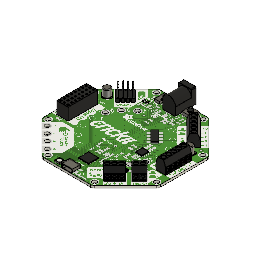
3093 Crickit CPX (Autodesk Fusion 360 design; units mm, degrees)
Autodesk Fusion 360 part; units mm, degrees
note: some values were not read from the file. Chosen so that the rebuilt part matches the saved one: which bodies a step acts on; which pieces of a blend or face edit are solid. Set by a fixed rule: which sketch regions a step uses.
(part 1 of 2)
sketch "cpx crickit" plane through (0, 0, 0) normal (0, 0, 1) x (1, 0, 0)
  arc A0 (-0.865, 37.0412) -> (-1.115, 36.7912) centre (-0.865, 36.7912) ccw
  arc A1 (2.385, 36.7912) -> (2.135, 37.0412) centre (2.135, 36.7912) ccw
  line L0 (16.3469, -40.64) -> (-16.3469, -40.64)
  line L1 (-4.3642, 34.692) -> (-3.915, 34.692)
  line L2 (-3.915, 31.692) -> (-4.3642, 31.692)
  arc A2 (-4.3642, 34.692) -> (-4.6142, 34.442) centre (-4.3642, 34.442) ccw
  arc A3 (-0.865, 30.7912) -> (-1.115, 30.592) centre (-0.8904, 30.5666) ccw
  arc A4 (40.64, 16.3469) -> (39.8961, 18.143) centre (38.1, 16.3469) ccw
  line L3 (-0.865, 37.0412) -> (2.135, 37.0412)
  line L4 (18.143, 39.8961) -> (39.8961, 18.143)
  arc A5 (2.135, 29.8928) -> (2.385, 30.092) centre (2.1604, 30.1174) ccw
  circle A6 centre (-9.779, 33.679) radius 0.5
  arc A7 (2.385, 30.592) -> (2.135, 30.7912) centre (2.1604, 30.5666) ccw
  arc A8 (-3.7158, 34.4674) -> (-3.915, 34.692) centre (-3.9277, 34.4801) ccw
  line L5 (-18.143, -39.8961) -> (-39.8961, -18.143)
  line L6 (2.135, 29.8928) -> (-0.865, 29.8928)
  arc A9 (18.143, 39.8961) -> (16.3469, 40.64) centre (16.3469, 38.1) ccw
  arc A10 (-3.915, 31.692) -> (-3.7158, 31.9674) centre (-3.9531, 31.9293) ccw
  line L7 (-1.115, 30.092) -> (-1.115, 30.592)
  line L8 (-0.865, 30.7912) -> (2.135, 30.7912)
  arc A11 (-4.6142, 31.942) -> (-4.3642, 31.692) centre (-4.3642, 31.942) ccw
  arc A12 (-1.115, 30.092) -> (-0.865, 29.8928) centre (-0.8904, 30.1174) ccw
  line L9 (4.05, -37.922) -> (4.05, -38.522)
  line L10 (-3.7158, 34.4674) -> (-3.7158, 31.9674)
  line L11 (-3.7, -37.572) -> (-3.5, -37.572)
  line L12 (2.385, 36.7912) -> (2.385, 36.3928)
  line L13 (40.64, 16.3469) -> (40.64, -16.3469)
  arc A13 (-4.05, -38.472) -> (-3.7, -38.872) centre (-3.675, -38.497) ccw
  arc A14 (3.6, -38.872) -> (4.05, -38.522) centre (3.65, -38.472) ccw
  circle A15 centre (-9.779, 36.679) radius 0.5
  arc A16 (-3.5, -38.872) -> (-3.15, -38.472) centre (-3.525, -38.497) ccw
  line L14 (-4.6142, 31.942) -> (-4.6142, 34.442)
  circle A17 centre (-1.95, -36.322) radius 0.35
  line L15 (-3.5, -38.872) -> (-3.7, -38.872)
  line L16 (-1.115, 36.3928) -> (-1.115, 36.7912)
  circle A18 centre (1.95, -36.322) radius 0.35
  line L17 (-39.8961, 18.143) -> (-18.143, 39.8961)
  arc A19 (2.135, 36.1428) -> (2.385, 36.3928) centre (2.135, 36.3928) ccw
  line L18 (-40.64, -16.3469) -> (-40.64, 16.3469)
  line L19 (3.15, -38.522) -> (3.15, -37.922)
  arc A20 (-39.8961, 18.143) -> (-40.64, 16.3469) centre (-38.1, 16.3469) ccw
  arc A21 (3.15, -38.522) -> (3.6, -38.872) centre (3.55, -38.472) ccw
  line L20 (2.135, 36.1428) -> (-0.865, 36.1428)
  line L21 (2.385, 30.592) -> (2.385, 30.092)
  arc A22 (-3.7, -37.572) -> (-4.05, -37.922) centre (-3.7, -37.922) ccw
  line L22 (-4.05, -38.472) -> (-4.05, -37.922)
  line L23 (39.8961, -18.143) -> (18.143, -39.8961)
  arc A23 (-1.115, 36.3928) -> (-0.865, 36.1428) centre (-0.865, 36.3928) ccw
  arc A24 (4.05, -37.922) -> (3.6, -37.572) centre (3.65, -37.972) ccw
  arc A25 (16.3469, -40.64) -> (18.143, -39.8961) centre (16.3469, -38.1) ccw
  line L24 (-16.3469, 40.64) -> (16.3469, 40.64)
  arc A26 (39.8961, -18.143) -> (40.64, -16.3469) centre (38.1, -16.3469) ccw
  arc A27 (-3.15, -37.922) -> (-3.5, -37.572) centre (-3.5, -37.922) ccw
  line L25 (-3.15, -37.922) -> (-3.15, -38.472)
  arc A28 (-16.3469, 40.64) -> (-18.143, 39.8961) centre (-16.3469, 38.1) ccw
  arc A29 (-18.143, -39.8961) -> (-16.3469, -40.64) centre (-16.3469, -38.1) ccw
  arc A30 (3.6, -37.572) -> (3.15, -37.922) centre (3.55, -37.972) ccw
  arc A31 (-40.64, -16.3469) -> (-39.8961, -18.143) centre (-38.1, -16.3469) ccw
  arc A32 (2.3241, -8.89) -> (1.4859, -8.89) centre (1.905, -8.89) ccw
  line L26 (1.985, 36.592) -> (-0.715, 36.592)
  arc A33 (16.129, 36.715) -> (16.129, 38.723) centre (16.129, 37.719) ccw
  arc A34 (-16.129, 38.723) -> (-16.129, 36.715) centre (-16.129, 37.719) ccw
  arc A35 (-16.129, 36.715) -> (-16.129, 38.723) centre (-16.129, 37.719) ccw
  arc A36 (3.3, -35.095) -> (3.3, -35.749) centre (3.3, -35.422) ccw
  arc A37 (37.719, 15.125) -> (37.719, 17.133) centre (37.719, 16.129) ccw
  arc A38 (-16.129, -38.723) -> (-16.129, -36.715) centre (-16.129, -37.719) ccw
  line L27 (-2.3935, -39.4285) -> (-2.3935, -37.0155)
  line L28 (2.3935, -39.4285) -> (4.8065, -39.4285)
  line L29 (-4.8065, -37.0155) -> (-4.8065, -39.4285)
  arc A39 (16.129, -38.723) -> (16.129, -36.715) centre (16.129, -37.719) ccw
  arc A40 (-16.129, -38.723) -> (-16.129, -36.715) centre (-16.129, -37.719) ccw
  arc A41 (37.719, 15.125) -> (37.719, 17.133) centre (37.719, 16.129) ccw
  line L30 (4.8065, -37.0155) -> (2.3935, -37.0155)
  arc A42 (-37.719, -17.133) -> (-37.719, -15.125) centre (-37.719, -16.129) ccw
  arc A43 (-37.719, -17.133) -> (-37.719, -15.125) centre (-37.719, -16.129) ccw
  arc A44 (1.985, 35.917) -> (1.985, 37.267) centre (1.985, 36.592) ccw
  arc A45 (16.129, 36.715) -> (16.129, 38.723) centre (16.129, 37.719) ccw
  line L31 (-3.3, -35.422) -> (-4.608, -35.422)
  arc A46 (37.719, -17.133) -> (37.719, -15.125) centre (37.719, -16.129) ccw
  line L32 (-2.3935, -37.0155) -> (-4.8065, -37.0155)
  arc A47 (37.719, -15.125) -> (37.719, -17.133) centre (37.719, -16.129) ccw
  line L33 (3.3, -35.422) -> (4.608, -35.422)
  arc A48 (-4.608, -35.095) -> (-4.608, -35.749) centre (-4.608, -35.422) ccw
  line L34 (2.3935, -39.4285) -> (4.8065, -39.4285)
  line L35 (-3.3, -35.422) -> (-4.608, -35.422)
  arc A49 (-16.129, 36.715) -> (-16.129, 38.723) centre (-16.129, 37.719) ccw
  arc A50 (16.129, 38.723) -> (16.129, 36.715) centre (16.129, 37.719) ccw
  arc A51 (-3.3, -35.749) -> (-3.3, -35.095) centre (-3.3, -35.422) ccw
  arc A52 (-3.3, -35.749) -> (-3.3, -35.095) centre (-3.3, -35.422) ccw
  arc A53 (-16.129, -36.715) -> (-16.129, -38.723) centre (-16.129, -37.719) ccw
  arc A54 (-0.715, 31.017) -> (-0.715, 29.667) centre (-0.715, 30.342) ccw
  line L36 (2.3935, -37.0155) -> (2.3935, -39.4285)
  line L37 (2.3935, -37.0155) -> (2.3935, -39.4285)
  arc A55 (37.719, 17.133) -> (37.719, 15.125) centre (37.719, 16.129) ccw
  line L38 (1.985, 36.592) -> (-0.715, 36.592)
  arc A56 (1.985, 29.667) -> (1.985, 31.017) centre (1.985, 30.342) ccw
  arc A57 (16.129, 38.723) -> (16.129, 36.715) centre (16.129, 37.719) ccw
  line L39 (4.8065, -37.0155) -> (2.3935, -37.0155)
  line L40 (-2.3935, -39.4285) -> (-2.3935, -37.0155)
  arc A58 (-3.49, 34.542) -> (-4.84, 34.542) centre (-4.165, 34.542) ccw
  line L41 (-4.8065, -39.4285) -> (-2.3935, -39.4285)
  arc A59 (-37.719, -15.125) -> (-37.719, -17.133) centre (-37.719, -16.129) ccw
  arc A60 (-37.719, 17.133) -> (-37.719, 15.125) centre (-37.719, 16.129) ccw
  arc A61 (-0.715, 31.017) -> (-0.715, 29.667) centre (-0.715, 30.342) ccw
  line L42 (-4.165, 34.542) -> (-4.165, 31.842)
  arc A62 (-4.84, 31.842) -> (-3.49, 31.842) centre (-4.165, 31.842) ccw
  arc A63 (-37.719, 15.125) -> (-37.719, 17.133) centre (-37.719, 16.129) ccw
  line L43 (4.8065, -39.4285) -> (4.8065, -37.0155)
  line L44 (-4.165, 34.542) -> (-4.165, 31.842)
  line L45 (-4.8065, -39.4285) -> (-2.3935, -39.4285)
  arc A64 (1.985, 35.917) -> (1.985, 37.267) centre (1.985, 36.592) ccw
  arc A65 (-37.719, 17.133) -> (-37.719, 15.125) centre (-37.719, 16.129) ccw
  arc A66 (37.719, 17.133) -> (37.719, 15.125) centre (37.719, 16.129) ccw
  arc A67 (16.129, -36.715) -> (16.129, -38.723) centre (16.129, -37.719) ccw
  arc A68 (1.4859, -8.89) -> (2.3241, -8.89) centre (1.905, -8.89) ccw
  arc A69 (-4.608, -35.095) -> (-4.608, -35.749) centre (-4.608, -35.422) ccw
  arc A70 (4.608, -35.749) -> (4.608, -35.095) centre (4.608, -35.422) ccw
  arc A71 (16.129, -36.715) -> (16.129, -38.723) centre (16.129, -37.719) ccw
  arc A72 (-16.129, 38.723) -> (-16.129, 36.715) centre (-16.129, 37.719) ccw
  line L46 (-2.3935, -37.0155) -> (-4.8065, -37.0155)
  arc A73 (37.719, -15.125) -> (37.719, -17.133) centre (37.719, -16.129) ccw
  arc A74 (3.3, -35.095) -> (3.3, -35.749) centre (3.3, -35.422) ccw
  arc A75 (-0.715, 37.267) -> (-0.715, 35.917) centre (-0.715, 36.592) ccw
  line L47 (1.985, 30.342) -> (-0.715, 30.342)
  arc A76 (-37.719, 15.125) -> (-37.719, 17.133) centre (-37.719, 16.129) ccw
  arc A77 (16.129, -38.723) -> (16.129, -36.715) centre (16.129, -37.719) ccw
  arc A78 (-3.49, 34.542) -> (-4.84, 34.542) centre (-4.165, 34.542) ccw
  line L48 (-4.8065, -37.0155) -> (-4.8065, -39.4285)
  arc A79 (37.719, -17.133) -> (37.719, -15.125) centre (37.719, -16.129) ccw
  arc A80 (-37.719, -15.125) -> (-37.719, -17.133) centre (-37.719, -16.129) ccw
  arc A81 (-0.715, 37.267) -> (-0.715, 35.917) centre (-0.715, 36.592) ccw
  line L49 (1.985, 30.342) -> (-0.715, 30.342)
  arc A82 (1.985, 29.667) -> (1.985, 31.017) centre (1.985, 30.342) ccw
  arc A83 (-4.84, 31.842) -> (-3.49, 31.842) centre (-4.165, 31.842) ccw
  arc A84 (1.4859, -8.89) -> (2.3241, -8.89) centre (1.905, -8.89) ccw
  arc A85 (-16.129, -36.715) -> (-16.129, -38.723) centre (-16.129, -37.719) ccw
  arc A86 (2.3241, -8.89) -> (1.4859, -8.89) centre (1.905, -8.89) ccw
  line L50 (4.8065, -39.4285) -> (4.8065, -37.0155)
  line L51 (3.3, -35.422) -> (4.608, -35.422)
  arc A87 (4.608, -35.749) -> (4.608, -35.095) centre (4.608, -35.422) ccw
  circle A88 centre (-21.844, 7.9248) radius 1.5
  circle A89 centre (-17.78, 14.859) radius 1.5
  circle A90 centre (-11.6332, 20.066) radius 1.5
  circle A91 centre (11.6332, -20.066) radius 1.5
  circle A92 centre (17.78, -14.859) radius 1.5
  circle A93 centre (21.844, -7.9248) radius 1.5
  circle A94 centre (18.7485, 28.6479) radius 0.635
  circle A95 centre (21.2233, 26.1731) radius 0.635
  circle A96 centre (23.6982, 23.6982) radius 0.635
  circle A97 centre (26.1731, 21.2233) radius 0.635
  circle A98 centre (28.6479, 18.7485) radius 0.635
  circle A99 centre (33.528, 7) radius 0.635
  circle A100 centre (33.528, 3.5) radius 0.635
  circle A101 centre (33.528, 0) radius 0.635
  circle A102 centre (33.528, -3.5) radius 0.635
  circle A103 centre (33.528, -7) radius 0.635
  circle A104 centre (27.7539, -20.5061) radius 0.635
  circle A105 centre (30.2288, -18.0312) radius 0.635
  circle A106 centre (17.8451, -30.4149) radius 0.635
  circle A107 centre (20.32, -27.94) radius 0.635
  circle A108 centre (22.7949, -25.4651) radius 0.635
  circle A109 centre (-36.068, 8.89) radius 0.635
  circle A110 centre (-33.528, 8.89) radius 0.635
  circle A111 centre (-30.988, 8.89) radius 0.635
  circle A112 centre (-36.068, 6.35) radius 0.635
  circle A113 centre (-33.528, 6.35) radius 0.635
  circle A114 centre (-30.988, 6.35) radius 0.635
  circle A115 centre (-36.068, 3.81) radius 0.635
  circle A116 centre (-33.528, 3.81) radius 0.635
  circle A117 centre (-30.988, 3.81) radius 0.635
  circle A118 centre (-36.068, 1.27) radius 0.635
  circle A119 centre (-33.528, 1.27) radius 0.635
  circle A120 centre (-30.988, 1.27) radius 0.635
  circle A121 centre (-36.068, -1.27) radius 0.635
  circle A122 centre (-33.528, -1.27) radius 0.635
  circle A123 centre (-30.988, -1.27) radius 0.635
  circle A124 centre (-36.068, -3.81) radius 0.635
  circle A125 centre (-33.528, -3.81) radius 0.635
  circle A126 centre (-30.988, -3.81) radius 0.635
  circle A127 centre (-36.068, -6.35) radius 0.635
  circle A128 centre (-33.528, -6.35) radius 0.635
  circle A129 centre (-30.988, -6.35) radius 0.635
  circle A130 centre (-36.068, -8.89) radius 0.635
  circle A131 centre (-33.528, -8.89) radius 0.635
  circle A132 centre (-30.988, -8.89) radius 0.635
  circle A133 centre (-34.1412, -20.2982) radius 1.5
  circle A134 centre (-29.3787, -24.9972) radius 1.5
  circle A135 centre (-24.8067, -29.5692) radius 1.5
  circle A136 centre (-20.1077, -34.2682) radius 1.5
  circle A137 centre (-22.8002, 28.1883) radius 0.635
  circle A138 centre (-24.5963, 26.3922) radius 0.635
  circle A139 centre (-26.3923, 24.5962) radius 0.635
  circle A140 centre (-28.1884, 22.8001) radius 0.635
  circle A141 centre (-21.0041, 26.3922) radius 0.635
  circle A142 centre (-22.8002, 24.5962) radius 0.635
  circle A143 centre (-24.5963, 22.8001) radius 0.635
  circle A144 centre (-26.3923, 21.0041) radius 0.635
  circle A145 centre (-19.2081, 24.5962) radius 0.635
  circle A146 centre (-21.0041, 22.8001) radius 0.635
  circle A147 centre (-22.8002, 21.0041) radius 0.635
  circle A148 centre (-24.5963, 19.208) radius 0.635
  dimension "d24" = 3
  dimension "d25" = 3
  dimension "d26" = 3
  dimension "d27" = 3
  dimension "d28" = 3
  dimension "d29" = 3
  dimension "d30" = 1.27
  dimension "d31" = 1.27
  dimension "d32" = 1.27
  dimension "d33" = 1.27
  dimension "d34" = 1.27
  dimension "d35" = 1.27
  dimension "d38" = 0
  dimension "d39" = -3.5
  dimension "d40" = 1.27
  dimension "d41" = 1.27
  dimension "d42" = 1.27
  dimension "d43" = 1.27
  dimension "d44" = 1.27
  dimension "d45" = 1.27
  dimension "d48" = 2.54
  dimension "d49" = -2.54
  dimension "d50" = 3
  dimension "d51" = 3
  dimension "d52" = 3
  dimension "d53" = 3
  dimension "d54" = 1.27
  dimension "d57" = -2.54
  dimension "d58" = -2.54
  measures "d24" diameter of A88
  measures "d25" diameter of A89
  measures "d26" diameter of A90
  measures "d27" diameter of A91
  measures "d28" diameter of A92
  measures "d29" diameter of A93
  measures "d30" diameter of A94
  measures "d31" diameter of A95
  measures "d32" diameter of A96
  measures "d33" diameter of A97
  measures "d34" diameter of A98
  measures "d35" diameter of A99
  measures "d40" diameter of A104
  measures "d41" diameter of A105
  measures "d42" diameter of A106
  measures "d43" diameter of A107
  measures "d44" diameter of A108
  measures "d45" diameter of A109
  measures "d50" diameter of A133
  measures "d51" diameter of A134
  measures "d52" diameter of A135
  measures "d53" diameter of A136
  measures "d54" diameter of A137
sketch "feather crickit" plane through (0, 0, 0) normal (0, 0, 1) x (1, 0, 0)
  circle A0 centre (-16.129, 37.719) radius 1.5
  arc A1 (39.8961, -18.143) -> (40.64, -16.3469) centre (38.1, -16.3469) ccw
  line L0 (40.64, 16.3469) -> (40.64, -16.3469)
  circle A2 centre (16.129, -37.719) radius 1.5
  arc A3 (-3.915, 31.692) -> (-3.7158, 31.9674) centre (-3.9531, 31.9293) ccw
  arc A4 (3.6, -38.872) -> (4.05, -38.522) centre (3.65, -38.472) ccw
  line L1 (-4.6142, 31.942) -> (-4.6142, 34.442)
  line L2 (4.064, -40.64) -> (3.683, -40.259)
  line L3 (-3.915, 31.692) -> (-4.3642, 31.692)
  arc A5 (-3.15, -37.922) -> (-3.5, -37.572) centre (-3.5, -37.922) ccw
  line L4 (3.15, -38.522) -> (3.15, -37.922)
  arc A6 (2.385, 36.7912) -> (2.135, 37.0412) centre (2.135, 36.7912) ccw
  line L5 (-4.3642, 34.692) -> (-3.915, 34.692)
  circle A7 centre (11.43, -17.78) radius 0.9
  line L6 (-0.865, 30.7912) -> (2.135, 30.7912)
  arc A8 (-4.05, -38.472) -> (-3.7, -38.872) centre (-3.675, -38.497) ccw
  circle A9 centre (1.95, -36.322) radius 0.35
  arc A10 (-0.865, 30.7912) -> (-1.115, 30.592) centre (-0.8904, 30.5666) ccw
  line L7 (18.143, 39.8961) -> (39.8961, 18.143)
  line L8 (-3.7158, 34.4674) -> (-3.7158, 31.9674)
  line L9 (4.05, -37.922) -> (4.05, -38.522)
  circle A11 centre (11.43, 17.78) radius 0.9
  line L10 (-4.05, -38.472) -> (-4.05, -37.922)
  circle A12 centre (-1.95, -36.322) radius 0.35
  arc A13 (40.64, 16.3469) -> (39.8961, 18.143) centre (38.1, 16.3469) ccw
  arc A14 (-40.64, -16.3469) -> (-39.8961, -18.143) centre (-38.1, -16.3469) ccw
  line L11 (-3.5, -38.872) -> (-3.7, -38.872)
  line L12 (2.385, 30.592) -> (2.385, 30.092)
  line L13 (-4.064, -40.64) -> (-16.3469, -40.64)
  arc A15 (-3.7, -37.572) -> (-4.05, -37.922) centre (-3.7, -37.922) ccw
  arc A16 (-0.865, 37.0412) -> (-1.115, 36.7912) centre (-0.865, 36.7912) ccw
  line L14 (-0.865, 37.0412) -> (2.135, 37.0412)
  line L15 (-3.7, -37.572) -> (-3.5, -37.572)
  arc A17 (-4.6142, 31.942) -> (-4.3642, 31.692) centre (-4.3642, 31.942) ccw
  line L16 (16.3469, -40.64) -> (4.064, -40.64)
  arc A18 (-1.115, 30.092) -> (-0.865, 29.8928) centre (-0.8904, 30.1174) ccw
  line L17 (-1.115, 36.3928) -> (-1.115, 36.7912)
  circle A19 centre (-11.43, 17.78) radius 0.9
  line L18 (-3.683, -40.259) -> (-4.064, -40.64)
  arc A20 (-1.115, 36.3928) -> (-0.865, 36.1428) centre (-0.865, 36.3928) ccw
  arc A21 (-39.8961, 18.143) -> (-40.64, 16.3469) centre (-38.1, 16.3469) ccw
  arc A22 (16.3469, -40.64) -> (18.143, -39.8961) centre (16.3469, -38.1) ccw
  arc A23 (-18.143, -39.8961) -> (-16.3469, -40.64) centre (-16.3469, -38.1) ccw
  arc A24 (2.135, 29.8928) -> (2.385, 30.092) centre (2.1604, 30.1174) ccw
  line L19 (39.8961, -18.143) -> (18.143, -39.8961)
  line L20 (2.385, 36.7912) -> (2.385, 36.3928)
  circle A25 centre (-9.779, 33.679) radius 0.5
  line L21 (-40.64, -16.3469) -> (-40.64, 16.3469)
  line L22 (2.135, 36.1428) -> (-0.865, 36.1428)
  arc A26 (2.385, 30.592) -> (2.135, 30.7912) centre (2.1604, 30.5666) ccw
  arc A27 (2.135, 36.1428) -> (2.385, 36.3928) centre (2.135, 36.3928) ccw
  circle A28 centre (-11.43, -7.62) radius 0.9
  line L23 (2.135, 29.8928) -> (-0.865, 29.8928)
  arc A29 (4.05, -37.922) -> (3.6, -37.572) centre (3.65, -37.972) ccw
  circle A30 centre (37.719, -16.129) radius 1.5
  arc A31 (3.6, -37.572) -> (3.15, -37.922) centre (3.55, -37.972) ccw
  arc A32 (3.15, -38.522) -> (3.6, -38.872) centre (3.55, -38.472) ccw
  line L24 (-3.15, -37.922) -> (-3.15, -38.472)
  circle A33 centre (-37.719, -16.129) radius 1.5
  line L25 (-39.8961, 18.143) -> (-18.143, 39.8961)
  line L26 (-18.143, -39.8961) -> (-39.8961, -18.143)
  arc A34 (-16.3469, 40.64) -> (-18.143, 39.8961) centre (-16.3469, 38.1) ccw
  circle A35 centre (16.129, 37.719) radius 1.5
  line L27 (3.683, -40.259) -> (-3.683, -40.259)
  arc A36 (-3.5, -38.872) -> (-3.15, -38.472) centre (-3.525, -38.497) ccw
  arc A37 (18.143, 39.8961) -> (16.3469, 40.64) centre (16.3469, 38.1) ccw
  circle A38 centre (-9.779, 36.679) radius 0.5
  arc A39 (-3.7158, 34.4674) -> (-3.915, 34.692) centre (-3.9277, 34.4801) ccw
  circle A40 centre (-16.129, -37.719) radius 1.5
  circle A41 centre (-37.719, 16.129) radius 1.5
  circle A42 centre (37.719, 16.129) radius 1.5
  line L28 (-16.3469, 40.64) -> (16.3469, 40.64)
  line L29 (-1.115, 30.092) -> (-1.115, 30.592)
  arc A43 (-4.3642, 34.692) -> (-4.6142, 34.442) centre (-4.3642, 34.442) ccw
  arc A44 (-5.715, -1.6891) -> (-5.715, -0.8509) centre (-5.715, -1.27) ccw
  arc A45 (-0.715, 31.017) -> (-0.715, 29.667) centre (-0.715, 30.342) ccw
  arc A46 (-5.715, 9.3091) -> (-5.715, 8.4709) centre (-5.715, 8.89) ccw
  arc A47 (-33.0835, -6.35) -> (-33.9725, -6.35) centre (-33.528, -6.35) ccw
  arc A48 (-33.9725, 1.27) -> (-33.0835, 1.27) centre (-33.528, 1.27) ccw
  arc A49 (-23.1145, 21.3184) -> (-22.4859, 20.6898) centre (-22.8002, 21.0041) ccw
  arc A50 (-28.5026, 23.1145) -> (-27.874, 22.4859) centre (-28.1883, 22.8002) ccw
  arc A51 (-5.715, 1.6891) -> (-5.715, 0.8509) centre (-5.715, 1.27) ccw
  arc A52 (-30.5435, -3.81) -> (-31.4325, -3.81) centre (-30.988, -3.81) ccw
  arc A53 (-33.0835, 6.35) -> (-33.9725, 6.35) centre (-33.528, 6.35) ccw
  arc A54 (29.0341, 19.1347) -> (28.2617, 18.3623) centre (28.6479, 18.7485) ccw
  arc A55 (5.715, 4.2291) -> (5.715, 3.3909) centre (5.715, 3.81) ccw
  arc A56 (5.715, -0.8509) -> (5.715, -1.6891) centre (5.715, -1.27) ccw
  arc A57 (28.2617, 18.3623) -> (29.0341, 19.1347) centre (28.6479, 18.7485) ccw
  arc A58 (-33.0835, -3.81) -> (-33.9725, -3.81) centre (-33.528, -3.81) ccw
  arc A59 (-24.0614, -28.8239) -> (-25.552, -30.3145) centre (-24.8067, -29.5692) ccw
  arc A60 (-5.715, -1.6891) -> (-5.715, -0.8509) centre (-5.715, -1.27) ccw
  arc A61 (-5.715, -4.2291) -> (-5.715, -3.3909) centre (-5.715, -3.81) ccw
  arc A62 (-5.715, 3.3909) -> (-5.715, 4.2291) centre (-5.715, 3.81) ccw
  arc A63 (-36.5125, -8.89) -> (-35.6235, -8.89) centre (-36.068, -8.89) ccw
  arc A64 (-5.715, -8.4709) -> (-5.715, -9.3091) centre (-5.715, -8.89) ccw
  arc A65 (32.9819, 3.5) -> (34.0741, 3.5) centre (33.528, 3.5) ccw
  arc A66 (-35.6235, 8.89) -> (-36.5125, 8.89) centre (-36.068, 8.89) ccw
  arc A67 (-5.715, -0.8509) -> (-5.715, -1.6891) centre (-5.715, -1.27) ccw
  line L30 (-4.8065, -37.0155) -> (-4.8065, -39.4285)
  arc A68 (-5.715, 0.8509) -> (-5.715, 1.6891) centre (-5.715, 1.27) ccw
  arc A69 (-31.4325, 1.27) -> (-30.5435, 1.27) centre (-30.988, 1.27) ccw
  line L31 (-3.3, -35.422) -> (-4.608, -35.422)
  arc A70 (-33.9725, 6.35) -> (-33.0835, 6.35) centre (-33.528, 6.35) ccw
  arc A71 (-19.5224, 24.9105) -> (-18.8938, 24.2819) centre (-19.2081, 24.5962) ccw
  arc A72 (-34.7595, -21.1705) -> (-33.2689, -19.6799) centre (-34.0142, -20.4252) ccw
  arc A73 (18.8595, -8.89) -> (19.7485, -8.89) centre (19.304, -8.89) ccw
  arc A74 (-31.4325, -6.35) -> (-30.5435, -6.35) centre (-30.988, -6.35) ccw
  arc A75 (29.0341, 19.1347) -> (28.2617, 18.3623) centre (28.6479, 18.7485) ccw
  arc A76 (-4.608, -35.095) -> (-4.608, -35.749) centre (-4.608, -35.422) ccw
  arc A77 (24.0844, 24.0844) -> (23.312, 23.312) centre (23.6982, 23.6982) ccw
  arc A78 (-5.715, -4.2291) -> (-5.715, -3.3909) centre (-5.715, -3.81) ccw
  arc A79 (24.0844, 24.0844) -> (23.312, 23.312) centre (23.6982, 23.6982) ccw
  arc A80 (-21.3184, 26.7066) -> (-20.6898, 26.078) centre (-21.0041, 26.3923) ccw
  arc A81 (18.2313, -30.8011) -> (17.4589, -30.0287) centre (17.8451, -30.4149) ccw
  arc A82 (5.715, -11.0109) -> (5.715, -11.8491) centre (5.715, -11.43) ccw
  arc A83 (21.6095, 26.5593) -> (20.8371, 25.7869) centre (21.2233, 26.1731) ccw
  arc A84 (34.0741, 0) -> (32.9819, 0) centre (33.528, 0) ccw
  line L32 (1.985, 30.342) -> (-0.715, 30.342)
  arc A85 (-22.4859, 27.874) -> (-23.1145, 28.5026) centre (-22.8002, 28.1883) ccw
  arc A86 (-5.715, 13.5509) -> (-5.715, 14.3891) centre (-5.715, 13.97) ccw
  arc A87 (-24.9105, 19.5224) -> (-24.2819, 18.8938) centre (-24.5962, 19.2081) ccw
  arc A88 (-33.9725, -6.35) -> (-33.0835, -6.35) centre (-33.528, -6.35) ccw
  arc A89 (-4.84, 31.842) -> (-3.49, 31.842) centre (-4.165, 31.842) ccw
  arc A90 (32.9819, -7) -> (34.0741, -7) centre (33.528, -7) ccw
  arc A91 (5.715, 0.8509) -> (5.715, 1.6891) centre (5.715, 1.27) ccw
  arc A92 (-33.9725, 3.81) -> (-33.0835, 3.81) centre (-33.528, 3.81) ccw
  line L33 (-3.3, -35.422) -> (-4.608, -35.422)
  line L34 (-2.3935, -39.4285) -> (-2.3935, -37.0155)
  arc A93 (-31.4325, -6.35) -> (-30.5435, -6.35) centre (-30.988, -6.35) ccw
  arc A94 (-20.6898, 26.078) -> (-21.3184, 26.7066) centre (-21.0041, 26.3923) ccw
  arc A95 (17.2085, -8.89) -> (16.3195, -8.89) centre (16.764, -8.89) ccw
  arc A96 (-26.078, 20.6898) -> (-26.7066, 21.3184) centre (-26.3923, 21.0041) ccw
  arc A97 (18.3623, 28.2617) -> (19.1347, 29.0341) centre (18.7485, 28.6479) ccw
  arc A98 (-36.5125, -8.89) -> (-35.6235, -8.89) centre (-36.068, -8.89) ccw
  line L35 (4.8065, -37.0155) -> (2.3935, -37.0155)
  arc A99 (-5.715, 6.7691) -> (-5.715, 5.9309) centre (-5.715, 6.35) ccw
  line L36 (-4.8065, -39.4285) -> (-2.3935, -39.4285)
  arc A100 (-20.6898, 26.078) -> (-21.3184, 26.7066) centre (-21.0041, 26.3923) ccw
  arc A101 (-33.0835, 6.35) -> (-33.9725, 6.35) centre (-33.528, 6.35) ccw
  arc A102 (-5.715, 6.7691) -> (-5.715, 5.9309) centre (-5.715, 6.35) ccw
  arc A103 (-5.715, 11.0109) -> (-5.715, 11.8491) centre (-5.715, 11.43) ccw
  arc A104 (-5.715, -9.3091) -> (-5.715, -8.4709) centre (-5.715, -8.89) ccw
  arc A105 (1.4859, -8.89) -> (2.3241, -8.89) centre (1.905, -8.89) ccw
  arc A106 (19.9338, -27.5538) -> (20.7062, -28.3262) centre (20.32, -27.94) ccw
  arc A107 (-35.6235, -6.35) -> (-36.5125, -6.35) centre (-36.068, -6.35) ccw
  arc A108 (-5.715, 0.8509) -> (-5.715, 1.6891) centre (-5.715, 1.27) ccw
  arc A109 (-4.84, 31.842) -> (-3.49, 31.842) centre (-4.165, 31.842) ccw
  arc A110 (-35.6235, 6.35) -> (-36.5125, 6.35) centre (-36.068, 6.35) ccw
  arc A111 (-30.5435, -6.35) -> (-31.4325, -6.35) centre (-30.988, -6.35) ccw
  arc A112 (28.2617, 18.3623) -> (29.0341, 19.1347) centre (28.6479, 18.7485) ccw
  arc A113 (-23.1145, 28.5026) -> (-22.4859, 27.874) centre (-22.8002, 28.1883) ccw
  arc A114 (-23.1145, 24.9105) -> (-22.4859, 24.2819) centre (-22.8002, 24.5962) ccw
  arc A115 (-35.6235, -6.35) -> (-36.5125, -6.35) centre (-36.068, -6.35) ccw
  arc A116 (23.1811, -25.8513) -> (22.4087, -25.0789) centre (22.7949, -25.4651) ccw
  arc A117 (-33.9725, -8.89) -> (-33.0835, -8.89) centre (-33.528, -8.89) ccw
  arc A118 (-33.0835, -6.35) -> (-33.9725, -6.35) centre (-33.528, -6.35) ccw
  arc A119 (-5.715, 8.4709) -> (-5.715, 9.3091) centre (-5.715, 8.89) ccw
  arc A120 (34.0741, 7) -> (32.9819, 7) centre (33.528, 7) ccw
  arc A121 (5.715, -9.3091) -> (5.715, -8.4709) centre (5.715, -8.89) ccw
  arc A122 (-33.0835, -3.81) -> (-33.9725, -3.81) centre (-33.528, -3.81) ccw
  arc A123 (-26.078, 24.2819) -> (-26.7066, 24.9105) centre (-26.3923, 24.5962) ccw
  arc A124 (-30.5435, 6.35) -> (-31.4325, 6.35) centre (-30.988, 6.35) ccw
  arc A125 (-5.715, -6.7691) -> (-5.715, -5.9309) centre (-5.715, -6.35) ccw
  arc A126 (18.2313, -30.8011) -> (17.4589, -30.0287) centre (17.8451, -30.4149) ccw
  arc A127 (5.715, -16.0909) -> (5.715, -16.9291) centre (5.715, -16.51) ccw
  arc A128 (-36.5125, 3.81) -> (-35.6235, 3.81) centre (-36.068, 3.81) ccw
  arc A129 (5.715, 6.7691) -> (5.715, 5.9309) centre (5.715, 6.35) ccw
  arc A130 (5.715, -18.6309) -> (5.715, -19.4691) centre (5.715, -19.05) ccw
  arc A131 (-31.4325, -8.89) -> (-30.5435, -8.89) centre (-30.988, -8.89) ccw
  arc A132 (-35.6235, -3.81) -> (-36.5125, -3.81) centre (-36.068, -3.81) ccw
  arc A133 (-36.5125, -6.35) -> (-35.6235, -6.35) centre (-36.068, -6.35) ccw
  arc A134 (26.5593, 21.6095) -> (25.7869, 20.8371) centre (26.1731, 21.2233) ccw
  arc A135 (32.9819, -3.5) -> (34.0741, -3.5) centre (33.528, -3.5) ccw
  arc A136 (34.0741, -3.5) -> (32.9819, -3.5) centre (33.528, -3.5) ccw
  arc A137 (1.985, 35.917) -> (1.985, 37.267) centre (1.985, 36.592) ccw
  arc A138 (-35.6235, -1.27) -> (-36.5125, -1.27) centre (-36.068, -1.27) ccw
  arc A139 (-18.8938, 24.2819) -> (-19.5224, 24.9105) centre (-19.2081, 24.5962) ccw
  arc A140 (-5.715, -5.9309) -> (-5.715, -6.7691) centre (-5.715, -6.35) ccw
  arc A141 (-31.4325, -1.27) -> (-30.5435, -1.27) centre (-30.988, -1.27) ccw
  arc A142 (-36.5125, 1.27) -> (-35.6235, 1.27) centre (-36.068, 1.27) ccw
  arc A143 (-23.1145, 24.9105) -> (-22.4859, 24.2819) centre (-22.8002, 24.5962) ccw
  arc A144 (16.3195, -8.89) -> (17.2085, -8.89) centre (16.764, -8.89) ccw
  arc A145 (20.8371, 25.7869) -> (21.6095, 26.5593) centre (21.2233, 26.1731) ccw
  line L37 (-4.165, 34.542) -> (-4.165, 31.842)
  arc A146 (32.9819, 7) -> (34.0741, 7) centre (33.528, 7) ccw
  arc A147 (-30.5435, -3.81) -> (-31.4325, -3.81) centre (-30.988, -3.81) ccw
  arc A148 (-5.715, 16.9291) -> (-5.715, 16.0909) centre (-5.715, 16.51) ccw
  arc A149 (22.4087, -25.0789) -> (23.1811, -25.8513) centre (22.7949, -25.4651) ccw
  arc A150 (-5.715, -9.3091) -> (-5.715, -8.4709) centre (-5.715, -8.89) ccw
  arc A151 (5.715, -13.5509) -> (5.715, -14.3891) centre (5.715, -13.97) ccw
  arc A152 (-30.5435, -8.89) -> (-31.4325, -8.89) centre (-30.988, -8.89) ccw
  arc A153 (2.3241, -8.89) -> (1.4859, -8.89) centre (1.905, -8.89) ccw
  arc A154 (5.715, -11.8491) -> (5.715, -11.0109) centre (5.715, -11.43) ccw
  arc A155 (5.715, 6.7691) -> (5.715, 5.9309) centre (5.715, 6.35) ccw
  arc A156 (5.715, 9.3091) -> (5.715, 8.4709) centre (5.715, 8.89) ccw
  arc A157 (-31.4325, -3.81) -> (-30.5435, -3.81) centre (-30.988, -3.81) ccw
  arc A158 (-34.7595, -21.1705) -> (-33.2689, -19.6799) centre (-34.0142, -20.4252) ccw
  arc A159 (5.715, 13.5509) -> (5.715, 14.3891) centre (5.715, 13.97) ccw
  line L38 (-4.165, 34.542) -> (-4.165, 31.842)
  line L39 (3.3, -35.422) -> (4.608, -35.422)
  line L40 (2.3935, -37.0155) -> (2.3935, -39.4285)
  arc A160 (18.8595, -8.89) -> (19.7485, -8.89) centre (19.304, -8.89) ccw
  arc A161 (-5.715, 13.5509) -> (-5.715, 14.3891) centre (-5.715, 13.97) ccw
  arc A162 (-5.715, -3.3909) -> (-5.715, -4.2291) centre (-5.715, -3.81) ccw
  arc A163 (-33.9725, -3.81) -> (-33.0835, -3.81) centre (-33.528, -3.81) ccw
  arc A164 (32.9819, 7) -> (34.0741, 7) centre (33.528, 7) ccw
  arc A165 (5.715, 16.0909) -> (5.715, 16.9291) centre (5.715, 16.51) ccw
  arc A166 (-5.715, 5.9309) -> (-5.715, 6.7691) centre (-5.715, 6.35) ccw
  arc A167 (5.715, -16.9291) -> (5.715, -16.0909) centre (5.715, -16.51) ccw
  arc A168 (-31.4325, -1.27) -> (-30.5435, -1.27) centre (-30.988, -1.27) ccw
  arc A169 (-33.0835, -1.27) -> (-33.9725, -1.27) centre (-33.528, -1.27) ccw
  arc A170 (2.3241, -8.89) -> (1.4859, -8.89) centre (1.905, -8.89) ccw
  arc A171 (-20.6898, 22.4859) -> (-21.3184, 23.1145) centre (-21.0041, 22.8002) ccw
  arc A172 (-5.715, -0.8509) -> (-5.715, -1.6891) centre (-5.715, -1.27) ccw
  arc A173 (-31.4325, 8.89) -> (-30.5435, 8.89) centre (-30.988, 8.89) ccw
  arc A174 (5.715, 3.3909) -> (5.715, 4.2291) centre (5.715, 3.81) ccw
  arc A175 (-5.715, 18.6309) -> (-5.715, 19.4691) centre (-5.715, 19.05) ccw
  arc A176 (-21.3184, 23.1145) -> (-20.6898, 22.4859) centre (-21.0041, 22.8002) ccw
  arc A177 (-30.5435, 6.35) -> (-31.4325, 6.35) centre (-30.988, 6.35) ccw
  arc A178 (-33.9725, 8.89) -> (-33.0835, 8.89) centre (-33.528, 8.89) ccw
  arc A179 (5.715, 8.4709) -> (5.715, 9.3091) centre (5.715, 8.89) ccw
  arc A180 (-35.6235, 1.27) -> (-36.5125, 1.27) centre (-36.068, 1.27) ccw
  arc A181 (-30.5435, 3.81) -> (-31.4325, 3.81) centre (-30.988, 3.81) ccw
  arc A182 (-33.0835, 8.89) -> (-33.9725, 8.89) centre (-33.528, 8.89) ccw
  arc A183 (25.7869, 20.8371) -> (26.5593, 21.6095) centre (26.1731, 21.2233) ccw
  arc A184 (-27.874, 22.4859) -> (-28.5026, 23.1145) centre (-28.1883, 22.8002) ccw
  arc A185 (20.7062, -28.3262) -> (19.9338, -27.5538) centre (20.32, -27.94) ccw
  arc A186 (-36.5125, -3.81) -> (-35.6235, -3.81) centre (-36.068, -3.81) ccw
  arc A187 (-33.0835, 3.81) -> (-33.9725, 3.81) centre (-33.528, 3.81) ccw
  arc A188 (-5.715, 14.3891) -> (-5.715, 13.5509) centre (-5.715, 13.97) ccw
  arc A189 (5.715, -5.9309) -> (5.715, -6.7691) centre (5.715, -6.35) ccw
  arc A190 (-24.9105, 23.1145) -> (-24.2819, 22.4859) centre (-24.5962, 22.8002) ccw
  arc A191 (-31.4325, 3.81) -> (-30.5435, 3.81) centre (-30.988, 3.81) ccw
  arc A192 (-36.5125, 6.35) -> (-35.6235, 6.35) centre (-36.068, 6.35) ccw
  arc A193 (34.0741, 7) -> (32.9819, 7) centre (33.528, 7) ccw
  arc A194 (-3.49, 34.542) -> (-4.84, 34.542) centre (-4.165, 34.542) ccw
  arc A195 (-5.715, 19.4691) -> (-5.715, 18.6309) centre (-5.715, 19.05) ccw
  arc A196 (-33.0835, -1.27) -> (-33.9725, -1.27) centre (-33.528, -1.27) ccw
  arc A197 (5.715, -11.0109) -> (5.715, -11.8491) centre (5.715, -11.43) ccw
  arc A198 (-5.715, 8.4709) -> (-5.715, 9.3091) centre (-5.715, 8.89) ccw
  line L41 (4.8065, -39.4285) -> (4.8065, -37.0155)
  arc A199 (-35.6235, -8.89) -> (-36.5125, -8.89) centre (-36.068, -8.89) ccw
  arc A200 (-5.715, 5.9309) -> (-5.715, 6.7691) centre (-5.715, 6.35) ccw
  arc A201 (-36.5125, -1.27) -> (-35.6235, -1.27) centre (-36.068, -1.27) ccw
  arc A202 (28.1401, -20.8923) -> (27.3677, -20.1199) centre (27.7539, -20.5061) ccw
  arc A203 (-33.9725, -6.35) -> (-33.0835, -6.35) centre (-33.528, -6.35) ccw
  arc A204 (-22.4859, 20.6898) -> (-23.1145, 21.3184) centre (-22.8002, 21.0041) ccw
  arc A205 (5.715, -5.9309) -> (5.715, -6.7691) centre (5.715, -6.35) ccw
  arc A206 (-33.0835, 3.81) -> (-33.9725, 3.81) centre (-33.528, 3.81) ccw
  arc A207 (34.0741, 3.5) -> (32.9819, 3.5) centre (33.528, 3.5) ccw
  arc A208 (1.985, 35.917) -> (1.985, 37.267) centre (1.985, 36.592) ccw
  arc A209 (5.715, -19.4691) -> (5.715, -18.6309) centre (5.715, -19.05) ccw
  arc A210 (-33.0835, 8.89) -> (-33.9725, 8.89) centre (-33.528, 8.89) ccw
  arc A211 (5.715, 16.0909) -> (5.715, 16.9291) centre (5.715, 16.51) ccw
  arc A212 (5.715, 19.4691) -> (5.715, 18.6309) centre (5.715, 19.05) ccw
  arc A213 (-28.6334, -24.2519) -> (-30.124, -25.7425) centre (-29.3787, -24.9972) ccw
  arc A214 (-20.853, -35.0135) -> (-19.3624, -33.5229) centre (-20.1077, -34.2682) ccw
  arc A215 (5.715, -8.4709) -> (5.715, -9.3091) centre (5.715, -8.89) ccw
  arc A216 (-5.715, 19.4691) -> (-5.715, 18.6309) centre (-5.715, 19.05) ccw
  arc A217 (-5.715, 16.0909) -> (-5.715, 16.9291) centre (-5.715, 16.51) ccw
  arc A218 (-5.715, 14.3891) -> (-5.715, 13.5509) centre (-5.715, 13.97) ccw
  arc A219 (-30.5435, 8.89) -> (-31.4325, 8.89) centre (-30.988, 8.89) ccw
  arc A220 (5.715, -6.7691) -> (5.715, -5.9309) centre (5.715, -6.35) ccw
  arc A221 (-31.4325, 6.35) -> (-30.5435, 6.35) centre (-30.988, 6.35) ccw
  arc A222 (34.0741, -3.5) -> (32.9819, -3.5) centre (33.528, -3.5) ccw
  arc A223 (5.715, -19.4691) -> (5.715, -18.6309) centre (5.715, -19.05) ccw
  arc A224 (16.3195, -8.89) -> (17.2085, -8.89) centre (16.764, -8.89) ccw
  arc A225 (23.1811, -25.8513) -> (22.4087, -25.0789) centre (22.7949, -25.4651) ccw
  arc A226 (5.715, 13.5509) -> (5.715, 14.3891) centre (5.715, 13.97) ccw
  arc A227 (19.1347, 29.0341) -> (18.3623, 28.2617) centre (18.7485, 28.6479) ccw
  arc A228 (5.715, -1.6891) -> (5.715, -0.8509) centre (5.715, -1.27) ccw
  arc A229 (-30.5435, 3.81) -> (-31.4325, 3.81) centre (-30.988, 3.81) ccw
  arc A230 (-5.715, 16.0909) -> (-5.715, 16.9291) centre (-5.715, 16.51) ccw
  arc A231 (-30.5435, -1.27) -> (-31.4325, -1.27) centre (-30.988, -1.27) ccw
  arc A232 (-26.7066, 21.3184) -> (-26.078, 20.6898) centre (-26.3923, 21.0041) ccw
  line L42 (-4.8065, -37.0155) -> (-4.8065, -39.4285)
  arc A233 (-5.715, 16.9291) -> (-5.715, 16.0909) centre (-5.715, 16.51) ccw
  arc A234 (28.1401, -20.8923) -> (27.3677, -20.1199) centre (27.7539, -20.5061) ccw
  line L43 (-2.3935, -39.4285) -> (-2.3935, -37.0155)
  arc A235 (-24.0614, -28.8239) -> (-25.552, -30.3145) centre (-24.8067, -29.5692) ccw
  arc A236 (32.9819, 0) -> (34.0741, 0) centre (33.528, 0) ccw
  arc A237 (-22.4859, 20.6898) -> (-23.1145, 21.3184) centre (-22.8002, 21.0041) ccw
  arc A238 (34.0741, 3.5) -> (32.9819, 3.5) centre (33.528, 3.5) ccw
  arc A239 (-24.2819, 26.078) -> (-24.9105, 26.7066) centre (-24.5962, 26.3923) ccw
  arc A240 (-31.4325, -3.81) -> (-30.5435, -3.81) centre (-30.988, -3.81) ccw
  arc A241 (-33.9725, 1.27) -> (-33.0835, 1.27) centre (-33.528, 1.27) ccw
  arc A242 (-36.5125, 6.35) -> (-35.6235, 6.35) centre (-36.068, 6.35) ccw
  arc A243 (-5.715, -5.9309) -> (-5.715, -6.7691) centre (-5.715, -6.35) ccw
  arc A244 (-36.5125, 8.89) -> (-35.6235, 8.89) centre (-36.068, 8.89) ccw
  arc A245 (-24.2819, 18.8938) -> (-24.9105, 19.5224) centre (-24.5962, 19.2081) ccw
  arc A246 (-5.715, 4.2291) -> (-5.715, 3.3909) centre (-5.715, 3.81) ccw
  arc A247 (5.715, -3.3909) -> (5.715, -4.2291) centre (5.715, -3.81) ccw
  arc A248 (3.3, -35.095) -> (3.3, -35.749) centre (3.3, -35.422) ccw
  arc A249 (-35.6235, 3.81) -> (-36.5125, 3.81) centre (-36.068, 3.81) ccw
  arc A250 (-30.124, -25.7425) -> (-28.6334, -24.2519) centre (-29.3787, -24.9972) ccw
  arc A251 (-28.5026, 23.1145) -> (-27.874, 22.4859) centre (-28.1883, 22.8002) ccw
  arc A252 (-19.3624, -33.5229) -> (-20.853, -35.0135) centre (-20.1077, -34.2682) ccw
  arc A253 (5.715, 18.6309) -> (5.715, 19.4691) centre (5.715, 19.05) ccw
  arc A254 (1.4859, -8.89) -> (2.3241, -8.89) centre (1.905, -8.89) ccw
  arc A255 (-21.3184, 23.1145) -> (-20.6898, 22.4859) centre (-21.0041, 22.8002) ccw
  arc A256 (-30.5435, 1.27) -> (-31.4325, 1.27) centre (-30.988, 1.27) ccw
  line L44 (1.985, 36.592) -> (-0.715, 36.592)
  arc A257 (-20.853, -35.0135) -> (-19.3624, -33.5229) centre (-20.1077, -34.2682) ccw
  arc A258 (-22.4859, 24.2819) -> (-23.1145, 24.9105) centre (-22.8002, 24.5962) ccw
  arc A259 (-4.608, -35.095) -> (-4.608, -35.749) centre (-4.608, -35.422) ccw
  arc A260 (34.0741, -7) -> (32.9819, -7) centre (33.528, -7) ccw
  arc A261 (-5.715, -6.7691) -> (-5.715, -5.9309) centre (-5.715, -6.35) ccw
  arc A262 (-0.715, 37.267) -> (-0.715, 35.917) centre (-0.715, 36.592) ccw
  arc A263 (25.7869, 20.8371) -> (26.5593, 21.6095) centre (26.1731, 21.2233) ccw
  arc A264 (-27.874, 22.4859) -> (-28.5026, 23.1145) centre (-28.1883, 22.8002) ccw
  arc A265 (-0.715, 37.267) -> (-0.715, 35.917) centre (-0.715, 36.592) ccw
  arc A266 (-23.1145, 28.5026) -> (-22.4859, 27.874) centre (-22.8002, 28.1883) ccw
  arc A267 (5.715, -8.4709) -> (5.715, -9.3091) centre (5.715, -8.89) ccw
  arc A268 (30.615, -18.4174) -> (29.8426, -17.645) centre (30.2288, -18.0312) ccw
  arc A269 (32.9819, 0) -> (34.0741, 0) centre (33.528, 0) ccw
  arc A270 (-21.3184, 26.7066) -> (-20.6898, 26.078) centre (-21.0041, 26.3923) ccw
  arc A271 (23.312, 23.312) -> (24.0844, 24.0844) centre (23.6982, 23.6982) ccw
  arc A272 (-5.715, 1.6891) -> (-5.715, 0.8509) centre (-5.715, 1.27) ccw
  arc A273 (-35.6235, -1.27) -> (-36.5125, -1.27) centre (-36.068, -1.27) ccw
  arc A274 (-5.715, 11.8491) -> (-5.715, 11.0109) centre (-5.715, 11.43) ccw
  arc A275 (-22.4859, 24.2819) -> (-23.1145, 24.9105) centre (-22.8002, 24.5962) ccw
  arc A276 (-5.715, 11.8491) -> (-5.715, 11.0109) centre (-5.715, 11.43) ccw
  arc A277 (-24.9105, 26.7066) -> (-24.2819, 26.078) centre (-24.5962, 26.3923) ccw
  arc A278 (-30.5435, -8.89) -> (-31.4325, -8.89) centre (-30.988, -8.89) ccw
  arc A279 (-36.5125, 1.27) -> (-35.6235, 1.27) centre (-36.068, 1.27) ccw
  arc A280 (-36.5125, -3.81) -> (-35.6235, -3.81) centre (-36.068, -3.81) ccw
  arc A281 (-19.5224, 24.9105) -> (-18.8938, 24.2819) centre (-19.2081, 24.5962) ccw
  arc A282 (-28.6334, -24.2519) -> (-30.124, -25.7425) centre (-29.3787, -24.9972) ccw
  arc A283 (5.715, 4.2291) -> (5.715, 3.3909) centre (5.715, 3.81) ccw
  arc A284 (5.715, 11.0109) -> (5.715, 11.8491) centre (5.715, 11.43) ccw
  arc A285 (-35.6235, 6.35) -> (-36.5125, 6.35) centre (-36.068, 6.35) ccw
  arc A286 (-33.9725, -1.27) -> (-33.0835, -1.27) centre (-33.528, -1.27) ccw
  arc A287 (-26.7066, 21.3184) -> (-26.078, 20.6898) centre (-26.3923, 21.0041) ccw
  arc A288 (23.312, 23.312) -> (24.0844, 24.0844) centre (23.6982, 23.6982) ccw
  line L45 (-2.3935, -37.0155) -> (-4.8065, -37.0155)
  arc A289 (34.0741, 0) -> (32.9819, 0) centre (33.528, 0) ccw
  arc A290 (5.715, 19.4691) -> (5.715, 18.6309) centre (5.715, 19.05) ccw
  arc A291 (-24.9105, 19.5224) -> (-24.2819, 18.8938) centre (-24.5962, 19.2081) ccw
  arc A292 (5.715, -18.6309) -> (5.715, -19.4691) centre (5.715, -19.05) ccw
  arc A293 (22.4087, -25.0789) -> (23.1811, -25.8513) centre (22.7949, -25.4651) ccw
  arc A294 (-26.7066, 24.9105) -> (-26.078, 24.2819) centre (-26.3923, 24.5962) ccw
  arc A295 (-3.3, -35.749) -> (-3.3, -35.095) centre (-3.3, -35.422) ccw
  arc A296 (-24.2819, 22.4859) -> (-24.9105, 23.1145) centre (-24.5962, 22.8002) ccw
  arc A297 (5.715, -0.8509) -> (5.715, -1.6891) centre (5.715, -1.27) ccw
  arc A298 (5.715, -14.3891) -> (5.715, -13.5509) centre (5.715, -13.97) ccw
  arc A299 (3.3, -35.095) -> (3.3, -35.749) centre (3.3, -35.422) ccw
  arc A300 (20.8371, 25.7869) -> (21.6095, 26.5593) centre (21.2233, 26.1731) ccw
  arc A301 (-30.5435, -1.27) -> (-31.4325, -1.27) centre (-30.988, -1.27) ccw
  arc A302 (-5.715, -3.3909) -> (-5.715, -4.2291) centre (-5.715, -3.81) ccw
  arc A303 (-0.715, 31.017) -> (-0.715, 29.667) centre (-0.715, 30.342) ccw
  arc A304 (5.715, 11.0109) -> (5.715, 11.8491) centre (5.715, 11.43) ccw
  arc A305 (-35.6235, -8.89) -> (-36.5125, -8.89) centre (-36.068, -8.89) ccw
  arc A306 (17.4589, -30.0287) -> (18.2313, -30.8011) centre (17.8451, -30.4149) ccw
  arc A307 (5.715, -13.5509) -> (5.715, -14.3891) centre (5.715, -13.97) ccw
  arc A308 (-24.2819, 26.078) -> (-24.9105, 26.7066) centre (-24.5962, 26.3923) ccw
  arc A309 (5.715, 18.6309) -> (5.715, 19.4691) centre (5.715, 19.05) ccw
  arc A310 (-35.6235, -3.81) -> (-36.5125, -3.81) centre (-36.068, -3.81) ccw
  arc A311 (-33.0835, 1.27) -> (-33.9725, 1.27) centre (-33.528, 1.27) ccw
  arc A312 (-33.0835, -8.89) -> (-33.9725, -8.89) centre (-33.528, -8.89) ccw
  arc A313 (-25.552, -30.3145) -> (-24.0614, -28.8239) centre (-24.8067, -29.5692) ccw
  arc A314 (-3.3, -35.749) -> (-3.3, -35.095) centre (-3.3, -35.422) ccw
  arc A315 (-33.9725, -3.81) -> (-33.0835, -3.81) centre (-33.528, -3.81) ccw
  arc A316 (29.8426, -17.645) -> (30.615, -18.4174) centre (30.2288, -18.0312) ccw
  arc A317 (5.715, -4.2291) -> (5.715, -3.3909) centre (5.715, -3.81) ccw
  arc A318 (5.715, 3.3909) -> (5.715, 4.2291) centre (5.715, 3.81) ccw
  arc A319 (-33.0835, 1.27) -> (-33.9725, 1.27) centre (-33.528, 1.27) ccw
  arc A320 (-31.4325, -8.89) -> (-30.5435, -8.89) centre (-30.988, -8.89) ccw
  arc A321 (-24.9105, 23.1145) -> (-24.2819, 22.4859) centre (-24.5962, 22.8002) ccw
  arc A322 (5.715, 5.9309) -> (5.715, 6.7691) centre (5.715, 6.35) ccw
  arc A323 (-35.6235, 3.81) -> (-36.5125, 3.81) centre (-36.068, 3.81) ccw
  arc A324 (-33.9725, 6.35) -> (-33.0835, 6.35) centre (-33.528, 6.35) ccw
  arc A325 (5.715, 16.9291) -> (5.715, 16.0909) centre (5.715, 16.51) ccw
  arc A326 (-33.0835, -8.89) -> (-33.9725, -8.89) centre (-33.528, -8.89) ccw
  arc A327 (17.4589, -30.0287) -> (18.2313, -30.8011) centre (17.8451, -30.4149) ccw
  arc A328 (1.985, 29.667) -> (1.985, 31.017) centre (1.985, 30.342) ccw
  arc A329 (5.715, -14.3891) -> (5.715, -13.5509) centre (5.715, -13.97) ccw
  line L46 (3.3, -35.422) -> (4.608, -35.422)
  arc A330 (-5.715, 4.2291) -> (-5.715, 3.3909) centre (-5.715, 3.81) ccw
  arc A331 (32.9819, 3.5) -> (34.0741, 3.5) centre (33.528, 3.5) ccw
  arc A332 (4.608, -35.749) -> (4.608, -35.095) centre (4.608, -35.422) ccw
  arc A333 (-35.6235, 8.89) -> (-36.5125, 8.89) centre (-36.068, 8.89) ccw
  arc A334 (-3.49, 34.542) -> (-4.84, 34.542) centre (-4.165, 34.542) ccw
  arc A335 (5.715, 0.8509) -> (5.715, 1.6891) centre (5.715, 1.27) ccw
  arc A336 (19.1347, 29.0341) -> (18.3623, 28.2617) centre (18.7485, 28.6479) ccw
  arc A337 (-31.4325, 6.35) -> (-30.5435, 6.35) centre (-30.988, 6.35) ccw
  arc A338 (26.5593, 21.6095) -> (25.7869, 20.8371) centre (26.1731, 21.2233) ccw
  arc A339 (-33.9725, -8.89) -> (-33.0835, -8.89) centre (-33.528, -8.89) ccw
  line L47 (1.985, 30.342) -> (-0.715, 30.342)
  arc A340 (-24.9105, 26.7066) -> (-24.2819, 26.078) centre (-24.5962, 26.3923) ccw
  line L48 (4.8065, -39.4285) -> (4.8065, -37.0155)
  arc A341 (5.715, 5.9309) -> (5.715, 6.7691) centre (5.715, 6.35) ccw
  arc A342 (21.6095, 26.5593) -> (20.8371, 25.7869) centre (21.2233, 26.1731) ccw
  arc A343 (-31.4325, 8.89) -> (-30.5435, 8.89) centre (-30.988, 8.89) ccw
  arc A344 (-5.715, 18.6309) -> (-5.715, 19.4691) centre (-5.715, 19.05) ccw
  arc A345 (32.9819, -3.5) -> (34.0741, -3.5) centre (33.528, -3.5) ccw
  arc A346 (-5.715, 3.3909) -> (-5.715, 4.2291) centre (-5.715, 3.81) ccw
  arc A347 (20.7062, -28.3262) -> (19.9338, -27.5538) centre (20.32, -27.94) ccw
  arc A348 (-26.078, 20.6898) -> (-26.7066, 21.3184) centre (-26.3923, 21.0041) ccw
  line L49 (-4.8065, -39.4285) -> (-2.3935, -39.4285)
  arc A349 (19.7485, -8.89) -> (18.8595, -8.89) centre (19.304, -8.89) ccw
  arc A350 (-5.715, -8.4709) -> (-5.715, -9.3091) centre (-5.715, -8.89) ccw
  arc A351 (-23.1145, 21.3184) -> (-22.4859, 20.6898) centre (-22.8002, 21.0041) ccw
  arc A352 (5.715, 11.8491) -> (5.715, 11.0109) centre (5.715, 11.43) ccw
  arc A353 (5.715, 11.8491) -> (5.715, 11.0109) centre (5.715, 11.43) ccw
  arc A354 (27.3677, -20.1199) -> (28.1401, -20.8923) centre (27.7539, -20.5061) ccw
  arc A355 (-5.715, 9.3091) -> (-5.715, 8.4709) centre (-5.715, 8.89) ccw
  arc A356 (17.2085, -8.89) -> (16.3195, -8.89) centre (16.764, -8.89) ccw
  arc A357 (18.3623, 28.2617) -> (19.1347, 29.0341) centre (18.7485, 28.6479) ccw
  arc A358 (-22.4859, 27.874) -> (-23.1145, 28.5026) centre (-22.8002, 28.1883) ccw
  arc A359 (5.715, -16.0909) -> (5.715, -16.9291) centre (5.715, -16.51) ccw
  arc A360 (32.9819, -7) -> (34.0741, -7) centre (33.528, -7) ccw
  arc A361 (-36.5125, 8.89) -> (-35.6235, 8.89) centre (-36.068, 8.89) ccw
  arc A362 (34.0741, -7) -> (32.9819, -7) centre (33.528, -7) ccw
  arc A363 (5.715, 9.3091) -> (5.715, 8.4709) centre (5.715, 8.89) ccw
  arc A364 (19.7485, -8.89) -> (18.8595, -8.89) centre (19.304, -8.89) ccw
  arc A365 (4.608, -35.749) -> (4.608, -35.095) centre (4.608, -35.422) ccw
  arc A366 (5.715, 1.6891) -> (5.715, 0.8509) centre (5.715, 1.27) ccw
  arc A367 (5.715, -4.2291) -> (5.715, -3.3909) centre (5.715, -3.81) ccw
  arc A368 (-36.5125, 3.81) -> (-35.6235, 3.81) centre (-36.068, 3.81) ccw
  arc A369 (5.715, -9.3091) -> (5.715, -8.4709) centre (5.715, -8.89) ccw
  line L50 (4.8065, -37.0155) -> (2.3935, -37.0155)
  arc A370 (-30.5435, 1.27) -> (-31.4325, 1.27) centre (-30.988, 1.27) ccw
  arc A371 (30.615, -18.4174) -> (29.8426, -17.645) centre (30.2288, -18.0312) ccw
  arc A372 (-24.2819, 22.4859) -> (-24.9105, 23.1145) centre (-24.5962, 22.8002) ccw
  arc A373 (-24.2819, 18.8938) -> (-24.9105, 19.5224) centre (-24.5962, 19.2081) ccw
  arc A374 (5.715, -1.6891) -> (5.715, -0.8509) centre (5.715, -1.27) ccw
  arc A375 (5.715, 16.9291) -> (5.715, 16.0909) centre (5.715, 16.51) ccw
  arc A376 (5.715, -11.8491) -> (5.715, -11.0109) centre (5.715, -11.43) ccw
  arc A377 (-5.715, 11.0109) -> (-5.715, 11.8491) centre (-5.715, 11.43) ccw
  arc A378 (5.715, 1.6891) -> (5.715, 0.8509) centre (5.715, 1.27) ccw
  arc A379 (5.715, -6.7691) -> (5.715, -5.9309) centre (5.715, -6.35) ccw
  arc A380 (5.715, 14.3891) -> (5.715, 13.5509) centre (5.715, 13.97) ccw
  arc A381 (5.715, -16.9291) -> (5.715, -16.0909) centre (5.715, -16.51) ccw
  arc A382 (-19.3624, -33.5229) -> (-20.853, -35.0135) centre (-20.1077, -34.2682) ccw
  arc A383 (27.3677, -20.1199) -> (28.1401, -20.8923) centre (27.7539, -20.5061) ccw
  arc A384 (-33.2689, -19.6799) -> (-34.7595, -21.1705) centre (-34.0142, -20.4252) ccw
  arc A385 (5.715, 8.4709) -> (5.715, 9.3091) centre (5.715, 8.89) ccw
  arc A386 (-20.6898, 22.4859) -> (-21.3184, 23.1145) centre (-21.0041, 22.8002) ccw
  arc A387 (-26.078, 24.2819) -> (-26.7066, 24.9105) centre (-26.3923, 24.5962) ccw
  arc A388 (-31.4325, 1.27) -> (-30.5435, 1.27) centre (-30.988, 1.27) ccw
  arc A389 (-18.8938, 24.2819) -> (-19.5224, 24.9105) centre (-19.2081, 24.5962) ccw
  arc A390 (-30.124, -25.7425) -> (-28.6334, -24.2519) centre (-29.3787, -24.9972) ccw
  arc A391 (-30.5435, -6.35) -> (-31.4325, -6.35) centre (-30.988, -6.35) ccw
  arc A392 (-30.5435, 8.89) -> (-31.4325, 8.89) centre (-30.988, 8.89) ccw
  arc A393 (29.8426, -17.645) -> (30.615, -18.4174) centre (30.2288, -18.0312) ccw
  line L51 (1.985, 36.592) -> (-0.715, 36.592)
  arc A394 (-33.9725, -1.27) -> (-33.0835, -1.27) centre (-33.528, -1.27) ccw
  arc A395 (-33.9725, 3.81) -> (-33.0835, 3.81) centre (-33.528, 3.81) ccw
  arc A396 (-31.4325, 3.81) -> (-30.5435, 3.81) centre (-30.988, 3.81) ccw
  line L52 (2.3935, -39.4285) -> (4.8065, -39.4285)
  line L53 (2.3935, -37.0155) -> (2.3935, -39.4285)
  arc A397 (-26.7066, 24.9105) -> (-26.078, 24.2819) centre (-26.3923, 24.5962) ccw
  arc A398 (-33.9725, 8.89) -> (-33.0835, 8.89) centre (-33.528, 8.89) ccw
  arc A399 (-33.2689, -19.6799) -> (-34.7595, -21.1705) centre (-34.0142, -20.4252) ccw
  line L54 (-2.3935, -37.0155) -> (-4.8065, -37.0155)
  arc A400 (5.715, 14.3891) -> (5.715, 13.5509) centre (5.715, 13.97) ccw
  arc A401 (-36.5125, -6.35) -> (-35.6235, -6.35) centre (-36.068, -6.35) ccw
  arc A402 (19.9338, -27.5538) -> (20.7062, -28.3262) centre (20.32, -27.94) ccw
  line L55 (2.3935, -39.4285) -> (4.8065, -39.4285)
  arc A403 (-35.6235, 1.27) -> (-36.5125, 1.27) centre (-36.068, 1.27) ccw
  arc A404 (-36.5125, -1.27) -> (-35.6235, -1.27) centre (-36.068, -1.27) ccw
  arc A405 (-25.552, -30.3145) -> (-24.0614, -28.8239) centre (-24.8067, -29.5692) ccw
  arc A406 (5.715, -3.3909) -> (5.715, -4.2291) centre (5.715, -3.81) ccw
  arc A407 (1.985, 29.667) -> (1.985, 31.017) centre (1.985, 30.342) ccw